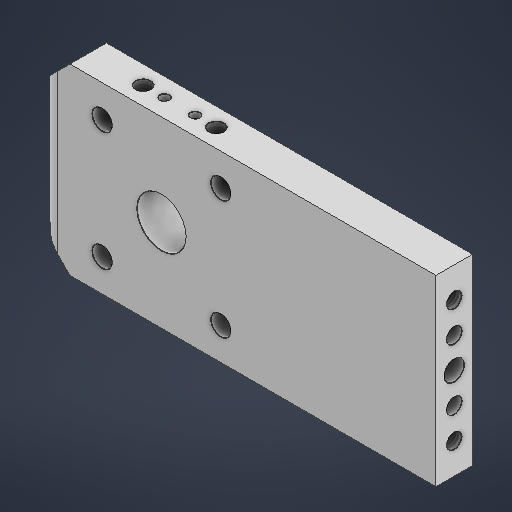
# Autodesk Inventor part: Standard
Saved by Autodesk Inventor 2025.4 (Build 294407000, 407)
## iProperties
Created: 2026-05-29
Part Number: Standard
Material: Generic
Document SubType Name: Modeling
Designer: VuQuan
Density: 1 g/cm^3
Appearance: Default
Author: VuQuan
Autodesk Inventor part; units mm, degrees
ref_plane "YZ Plane" through (0, 0, 0) normal (1, 0, 0) x (0, 1, 0)
ref_plane "XZ Plane" through (0, 0, 0) normal (0, 1, 0) x (-1, 0, 0)
ref_plane "XY Plane" through (0, 0, 0) normal (0, 0, 1) x (1, 0, 0)
sketch "Sketch1" plane through (0, 0, 0) normal (0, 0, 1) x (1, 0, 0)
  line L0 (-60, 30) -> (60, 30)
  line L1 (60, 30) -> (60, -30)
  line L2 (60, -30) -> (-60, -30)
  line L3 (-70, -20) -> (-70, 20)
  line L4 (-60, 30) -> (-70, 20)
  line L5 (-70, -20) -> (-60, -30)
  circle A0 centre (-30, 0) radius 27.5 construction
  circle A1 centre (-49.4454, 19.4454) radius 3.25
  line L6 (-30, 0) -> (-49.4454, 19.4454) construction
  line L7 (0, 0) -> (-30, 0) construction
  circle A2 centre (-49.4454, -19.4454) radius 3.25
  circle A3 centre (-10.5546, -19.4454) radius 3.25
  circle A4 centre (-10.5546, 19.4454) radius 3.25
  circle A5 centre (-30, 0) radius 8
  circle A6 centre (-15, 0) radius 5.5
  circle A7 centre (-15, 0) radius 3.25
  line L8 (-30, 0) -> (-30, 30) construction
  point P0 (-70, 30)
  point P1 (-70, -30)
  point P2 (0, 30)
  point P3 (-70, 0)
  point P4 (60, 0)
  point P5 (60, 10)
  point P6 (60, 20)
  point P7 (60, -10)
  point P8 (60, -20)
  point P9 (-35, 30)
  point P10 (-42, 30)
  point P11 (-25, 30)
  point P12 (-18, 30)
  dimension "d6" = 55
  dimension "d0" = 10
  dimension "d1" = 10
  dimension "d2" = 10
  dimension "d3" = 10
  dimension "d4" = 60
  dimension "d5" = 130
  dimension "d7" = 90
  dimension "d8" = 6.5
  dimension "d9" = 45
  dimension "d12" = 360
  dimension "d14" = 16
  dimension "d15" = 10
  dimension "d16" = 20
  dimension "d17" = 11
  dimension "d18" = 6.5
  dimension "d19" = 75
  dimension "d20" = 10
  dimension "d21" = 24
  constraints: 18 end point, 9 point on line, 7 centre point, 4 midpoint, 4 symmetric about line, 2 coincident, 2 horizontal, 2 horizontal alignment, 2 parallel, 2 perpendicular, 1 vertical alignment, 12 other
  measures "d0" distance of L0.start point (-70, 30)
  measures "d1" distance of L3.end point (-70, 30)
  measures "d2" distance of L3.start point (-70, -30)
  measures "d3" distance of L2.end point (-70, -30)
  measures "d4" distance between parallel lines of L2 L0
  measures "d5" distance between parallel lines of L1 L3
  measures "d7" distance from line of L1 L6.start
  measures "d8" diameter of A1
  measures "d9" angle of L7 L6
  measures "d14" diameter of A5
  measures "d15" distance of point (60, 20) point (60, 10)
  measures "d16" diameter of point (60, 10) L7
  measures "d17" diameter of A6
  measures "d18" diameter of A7
  measures "d19" distance from line of L1 A6.centre
  measures "d20" diameter of point (-35, 30) L8
  measures "d21" diameter of point (-42, 30) L8
extrude "Extrusion1" add sketch "Sketch1" along normal mid plane 12 contours L0 L1 L2 L5 L3 L4 | A6 | A7
extrude "Extrusion2" cut sketch "Sketch1" along normal mid plane 1.5 from surface at -6 contours A6 | A7
sketch "Sketch2" plane through (60, -30, 6) normal (1, 0, 0) x (0, 0, -1)
  point P0 (6, 30)
  point P1 (6, 20)
  point P2 (6, 30)
  point P3 (6, 40)
  point P4 (6, 50)
  point P5 (6, 10)
hole "Hole1" at (60, 10, 0) at (60, -10, 0) direction (-1, 0, 0) diameter 5 depth 15 tip angle 118
hole "Hole2" at (60, -20, 0) at (60, 20, 0) direction (-1, 0, 0) diameter 4.917 depth 20 tip angle 118 thread size "M6x1" class "6H" standard "ISO Metric profile"
hole "Hole3" at (60, 0, 0) direction (-1, 0, 0) diameter 6.5 depth 78.5 tip angle 118
sketch "Sketch3" plane through (-15, 0, -5.25) normal (0, 0, -1) x (-1, 0, 0)
  circle A0 centre (0, 0) radius 5.5 projected
  point P0 (-15, 0)
  constraints: 1 coincident
hole "Hole4" at (-15, 0, -5.25) direction (0, 0, 1) diameter 6.5 end up to surface
sketch "Sketch4" plane through (-60, 30, 6) normal (0, 1, 0) x (1, 0, 0)
  point P0 (60, 6)
  point P1 (42, 6)
  point P2 (35, 6)
  point P3 (25, 6)
  point P4 (18, 6)
hole "Hole5" at (-42, 30, 0) at (-18, 30, 0) direction (0, -1, 0) diameter 4.917 depth 20 tip angle 118 thread size "M6x1" class "6H" standard "ISO Metric profile"
hole "Hole6" at (-25, 30, 0) at (-35, 30, 0) direction (0, -1, 0) diameter 3 depth 12 tip angle 118
fillet "Fillet1" radius 6 2 edges at (-70, 0, 6) (-70, 0, -6)
chamfer "Chamfer2" distance 0.1 angle 45 19 edges at (-38, 0, 6) (-38, 0, -6) (-52.6954, -19.4454, 6) (-13.8046, -19.4454, 6) (-13.8046, 19.4454, 6) (-52.6954, 19.4454, 6) (-13.8046, 19.4454, -6) (-52.6954, 19.4454, -6) (-13.8046, -19.4454, -6) (-52.6954, -19.4454, -6) (-18, 30, -2.4585) (-25, 30, -1.5) (-35, 30, -1.5) (-42, 30, -2.4585) (60, 20, 2.4585) (60, 10, 2.5) (60, 0, 3.25) (60, -10, 2.5) (60, -20, 2.4585)
equation "\"d1\" = d0"
equation "\"d2\" = d0"
equation "\"d3\" = d2"
body "Solid1"
